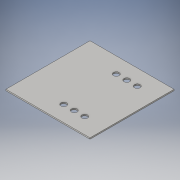
# Autodesk Inventor part: Slider
Saved by Autodesk Inventor 2016 (Build 200138000, 138)
## iProperties
Created: 2015-11-12
Part Number: Slider
Material: Generic
Document SubType Name: Modeling
Designer: Rachel
Density: 1 g/cm^3
Appearance: Default
Author: Rachel
Autodesk Inventor part; units mm, degrees
ref_plane "YZ Plane" through (0, 0, 0) normal (1, 0, 0) x (0, 1, 0)
ref_plane "XZ Plane" through (0, 0, 0) normal (0, 1, 0) x (-1, 0, 0)
ref_plane "XY Plane" through (0, 0, 0) normal (0, 0, 1) x (1, 0, 0)
sketch "Sketch1" plane through (0, 0, 0) normal (0, 1, 0) x (-1, 0, 0)
  line L0 (41.656, 38.862) -> (-59.944, 38.862)
  line L1 (-59.944, 38.862) -> (-59.944, -62.738)
  line L2 (-59.944, -62.738) -> (41.656, -62.738)
  line L3 (41.656, -62.738) -> (41.656, 38.862)
  circle A0 centre (-9.144, 19.812) radius 3.429
  circle A1 centre (-21.844, 19.812) radius 3.429
  circle A2 centre (-34.544, 19.812) radius 3.429
  circle A3 centre (-9.144, -43.688) radius 3.429
  circle A4 centre (-21.844, -43.688) radius 3.429
  circle A5 centre (-34.544, -43.688) radius 3.429
  point P0 (0, 0)
  point P1 (-9.144, 19.812)
  point P2 (-9.144, -43.688)
  point P3 (-9.144, -43.688)
  dimension "d0" = 101.6
  dimension "d1" = 101.6
  dimension "d3" = 6.858
  dimension "d4" = 12.7
  dimension "d5" = 12.7
  dimension "d6" = 25.4
  dimension "d8" = 19.05
  dimension "d9" = 19.05
  dimension "d10" = 6.858
  dimension "d11" = 12.7
  dimension "d12" = 12.7
  constraints: 8 end point, 6 centre point, 4 equal radius, 2 parallel, 1 horizontal, 1 perpendicular
  measures "d0" distance of L2.end L0.start
  measures "d1" distance of L1.end L2.end
  measures "d3" diameter of A0
  measures "d4" distance of A1.centre A0.centre
  measures "d5" distance of A1.centre A2.centre
  measures "d6" distance from line of L1 A2.centre
  measures "d8" distance from line of L0 point (-9.144, 19.812)
  measures "d9" distance from line of L2 point (-9.144, -43.688)
  measures "d10" diameter of A3
  measures "d11" distance of A4.centre A3.centre
  measures "d12" distance of A4.centre A5.centre
extrude "Extrusion1" add sketch "Sketch1" along normal blind 1.5875
body "Solid1"
